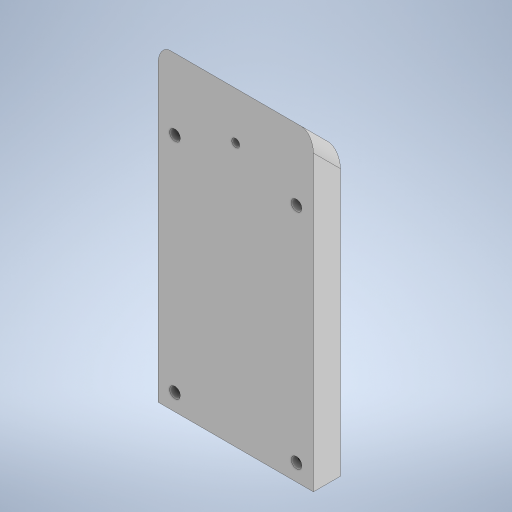
# Autodesk Inventor part: Bauteil unten
Saved by Autodesk Inventor 2024 (Build 280153000, 153)
## iProperties
Created: 2025-04-06
Part Number: Bauteil unten
Material: Generisch
Document SubType Name: Modeling
Designer: fynnb
Density: 1 g/cm^3
Appearance: Vorgabe
Mass: 466.132 g
Surface Area: 748.117 cm^2
Volume: 466.132 cm^3
Author: fynnb
Autodesk Inventor part; units mm, degrees
ref_plane "YZ Plane" through (0, 0, 0) normal (1, 0, 0) x (0, 1, 0)
ref_plane "XZ Plane" through (0, 0, 0) normal (0, 1, 0) x (-1, 0, 0)
ref_plane "XY Plane" through (0, 0, 0) normal (0, 0, 1) x (1, 0, 0)
sketch "Skizze1" plane through (0, 0, 0) normal (0, 1, 0) x (-1, 0, 0)
  line L0 (50.5319, 87.7571) -> (-64.4681, 87.7571)
  line L1 (-64.4681, 87.7571) -> (-64.4681, -102.2429)
  line L2 (-64.4681, -102.2429) -> (50.5319, -102.2429)
  line L3 (50.5319, -102.2429) -> (50.5319, 87.7571)
  point P0 (0, 0)
  dimension "d0" = 190
  dimension "d1" = 115
  constraints: 8 end point, 2 parallel, 1 horizontal, 1 perpendicular
  measures "d0" distance of L2.end L0.start
  measures "d1" distance of L1.end L2.end
extrude "Extrusion1" add sketch "Skizze1" along normal blind 20
sketch "Skizze2" plane through (0, 20, 0) normal (0, 1, 0) x (1, 0, 0)
  line L0 (-50.5319, 102.2429) -> (-50.5319, -87.7571) projected
  line L1 (64.4681, -87.7571) -> (64.4681, 102.2429) projected
  line L2 (-50.5319, -87.7571) -> (64.4681, -87.7571) projected
  line L3 (64.4681, 102.2429) -> (-50.5319, 102.2429) projected
  point P0 (0, 0)
  point P1 (-38.0319, 89.7569)
  point P2 (-38.0319, -75.2431)
  point P3 (51.9681, -75.2431)
  point P4 (51.9681, 89.7569)
  point P5 (-50.5319, 90.2429)
  point P6 (-50.5319, -75.7571)
  point P7 (64.4681, -75.7571)
  point P8 (64.4681, 90.2429)
  point P9 (-38.5319, -87.7571)
  point P10 (52.4681, -87.7571)
  point P11 (52.4681, 102.2429)
  point P12 (-38.5319, 102.2429)
  dimension "d6" = 12.5
  dimension "d8" = 12.5
  dimension "d9" = 12.5
  dimension "d12" = 12.5
  dimension "d24" = 12.514
  dimension "d25" = 12.514
  dimension "d26" = 12.486
  dimension "d27" = 12.486
  measures "d6" distance from line of L0 point (-38.032, 89.757)
  measures "d8" distance from line of L0 point (-38.032, -75.243)
  measures "d9" distance from line of L1 point (51.968, -75.243)
  measures "d12" distance from line of L1 point (51.968, 89.757)
  measures "d24" distance from line of L2 point (-38.032, -75.243)
  measures "d25" distance from line of L2 point (51.968, -75.243)
  measures "d26" distance from line of L3 point (-38.032, 89.757)
  measures "d27" distance from line of L3 point (51.968, 89.757)
hole "Bohrung1" at (-38.0319, 20, -89.7569) at (-38.0319, 20, 75.2431) at (51.9681, 20, 75.2431) at (51.9681, 20, -89.7569) direction (0, -1, 0) diameter 8 depth 20
sketch "Skizze5" plane through (64.4681, 0, -102.2429) normal (0, 0, -1) x (-1, 0, 0)
  line L0 (115, 0) -> (115, 20) projected
  line L1 (0, 20) -> (115, 20) projected
  line L2 (0, 0) -> (0, 20) projected
  point P0 (64.4681, 0)
  point P1 (98.75, 7.5)
  point P2 (73.75, 7.5)
  point P3 (41.25, 7.5)
  point P4 (16.25, 7.5)
  dimension "d33" = 25
  dimension "d34" = 25
  dimension "d35" = 32.5
  dimension "d36" = 12.5
  dimension "d55" = 16.25
  dimension "d56" = 16.25
  measures "d33" distance of point (98.75, 7.5) point (73.75, 7.5)
  measures "d34" distance of point (16.25, 7.5) point (41.25, 7.5)
  measures "d35" distance of point (41.25, 7.5) point (73.75, 7.5)
  measures "d36" distance from line of L1 point (41.25, 7.5)
  measures "d55" distance from line of L2 point (16.25, 7.5)
  measures "d56" distance from line of L0 point (98.75, 7.5)
hole "Bohrung2" at (-34.2819, 7.5, -102.2429) at (-9.2819, 7.5, -102.2429) at (23.2181, 7.5, -102.2429) at (48.2181, 7.5, -102.2429) direction (0, 0, 1) diameter 5.3 depth 20
sketch "Skizze6" plane through (0, 20, 0) normal (0, 1, 0) x (1, 0, 0)
  line L0 (-23.0319, 12.2429) -> (36.9681, 12.2429)
  line L1 (36.9681, 12.2429) -> (36.9681, 77.2429)
  line L2 (36.9681, 77.2429) -> (-23.0319, 77.2429)
  line L3 (-23.0319, 77.2429) -> (-23.0319, 12.2429)
  line L4 (-50.5319, 102.2429) -> (-50.5319, -87.7571) projected
  line L5 (64.4681, 102.2429) -> (-50.5319, 102.2429) projected
  point P0 (0, 0)
  dimension "d44" = 65
  dimension "d45" = 60
  dimension "d46" = 27.5
  dimension "d47" = 25
  constraints: 8 end point, 2 parallel, 1 horizontal, 1 perpendicular
  measures "d44" distance of L2.end L0.start
  measures "d45" distance of L1.end L2.end
  measures "d46" distance between parallel lines of L3 L4
  measures "d47" distance between parallel lines of L5 L2
extrude "Extrusion2" add sketch "Skizze6" along normal blind 10
fillet "Rundung3" radius 9 1 edges at (6.9681, 30, -12.2429)
sketch "Skizze7" plane through (-50.5319, 0, 87.7571) normal (0, 0, 1) x (1, 0, 0)
  line L0 (0, 0) -> (115, 0) projected
  line L1 (0, 20) -> (115, 20) projected
  line L2 (115, 0) -> (0, 0)
  line L3 (0, 0) -> (0, 20)
  line L4 (0, 20) -> (115, 20)
  line L5 (115, 20) -> (115, 0)
  point P0 (50.5319, 0)
  constraints: 8 end point, 2 parallel, 1 horizontal, 1 perpendicular
extrude "Extrusion3" add sketch "Skizze7" along normal blind 40
sketch "Skizze8" plane through (-50.5319, 0, -102.2429) normal (-1, 0, 0) x (0, 0, 1)
  line L0 (230, 20) -> (230, 0) projected
  line L1 (230, 20) -> (210, 20)
  line L2 (0, 20) -> (230, 20) projected
  line L3 (230, 20) -> (230, 0)
  line L4 (210, 20) -> (230, 0)
  point P0 (102.2429, 0)
  dimension "d60" = 20
  constraints: 6 end point, 1 collinear, 1 point on line
  measures "d60" distance of L0.start L1.end
extrude "Extrusion4" cut sketch "Skizze8" against normal through all
fillet "Rundung5" radius 9 2 edges at (-50.5319, 10, 117.7571) (64.4681, 10, 117.7571)
sketch "Skizze11" plane through (0, 20, 0) normal (0, 1, 0) x (1, 0, 0)
  line L0 (-50.5319, 102.2429) -> (-50.5319, -95.0292) projected
  line L1 (-41.5319, -107.7571) -> (55.4681, -107.7571) projected
  point P0 (0, 0)
  point P1 (6.9681, -92.7571)
  dimension "d65" = 57.5
  dimension "d66" = 15
  measures "d65" distance from line of L0 point (6.968, -92.757)
  measures "d66" distance from line of L1 point (6.968, -92.757)
hole "Bohrung3" at (6.9681, 20, 92.7571) direction (0, -1, 0) diameter 6 end through all
sketch "Skizze12" plane through (0, 20, 0) normal (0, 1, 0) x (1, 0, 0)
  line L0 (-30.0319, -87.7571) -> (43.9681, -87.7571)
  line L1 (43.9681, -87.7571) -> (43.9681, 2.2429)
  line L2 (43.9681, 2.2429) -> (-30.0319, 2.2429)
  line L3 (-30.0319, 2.2429) -> (-30.0319, -87.7571)
  line L4 (-50.5319, 102.2429) -> (-50.5319, -95.0292) projected
  line L5 (-41.5319, -107.7571) -> (55.4681, -107.7571) projected
  point P0 (0, 0)
  dimension "d74" = 90
  dimension "d75" = 74
  dimension "d76" = 20.5
  dimension "d77" = 20
  constraints: 8 end point, 2 parallel, 1 horizontal, 1 perpendicular
  measures "d74" distance between parallel lines of L2 L0
  measures "d75" distance between parallel lines of L1 L3
  measures "d76" distance between parallel lines of L4 L3
  measures "d77" distance between parallel lines of L5 L0
extrude "Extrusion5" cut sketch "Skizze12" against normal blind 10
sketch "Skizze13" plane through (0, 20, 0) normal (0, 1, 0) x (1, 0, 0)
  circle A0 centre (-38.0319, -75.2431) radius 4 projected
  circle A1 centre (-38.0319, -75.2431) radius 7
  circle A2 centre (51.9681, -75.2431) radius 4 projected
  circle A3 centre (51.9681, -75.2431) radius 7
  circle A4 centre (-38.0319, 89.7569) radius 4 projected
  circle A5 centre (-38.0319, 89.7569) radius 7
  circle A6 centre (51.9681, 89.7569) radius 4 projected
  circle A7 centre (51.9681, 89.7569) radius 7
  point P0 (0, 0)
  dimension "d80" = 14
  dimension "d81" = 14
  dimension "d82" = 14
  dimension "d83" = 14
  constraints: 4 centre point, 4 coincident
  measures "d80" diameter of A1
  measures "d81" diameter of A3
  measures "d82" diameter of A5
  measures "d83" diameter of A7
extrude "Extrusion6" cut sketch "Skizze13" against normal blind 4 contours A0 | A1 | A2 | A3 | A4 | A5 | A6 | A7
